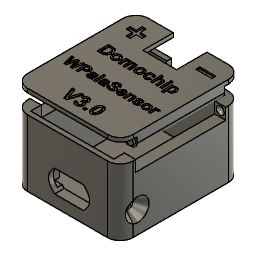
WPalaSensor v12 (Autodesk Fusion 360 design; units mm, degrees)
Autodesk Fusion 360 part; units mm, degrees
form "Form1" [no effect]
sketch "Bases" plane through (0, 0, 0) normal (0, 1, 0) x (1, 0, 0)
  line L0 (7.8348, 4.0595) -> (32.8348, 4.0595)
  line L1 (36.8348, 8.0595) -> (36.8348, 37.8595)
  line L2 (32.8348, 41.8595) -> (7.8348, 41.8595)
  line L3 (3.8348, 37.8595) -> (3.8348, 8.0595)
  arc A0 (7.8348, 41.8595) -> (3.8348, 37.8595) centre (7.8348, 37.8595) ccw
  arc A1 (36.8348, 37.8595) -> (32.8348, 41.8595) centre (32.8348, 37.8595) ccw
  arc A2 (32.8348, 4.0595) -> (36.8348, 8.0595) centre (32.8348, 8.0595) ccw
  arc A3 (3.8348, 8.0595) -> (7.8348, 4.0595) centre (7.8348, 8.0595) ccw
  arc A4 (3.8348, 8.0595) -> (7.8348, 4.0595) centre (7.8348, 8.0595) ccw
  arc A5 (32.8348, 4.0595) -> (36.8348, 8.0595) centre (32.8348, 8.0595) ccw
  line L4 (3.8348, 37.8595) -> (3.8348, 8.0595)
  line L5 (36.8348, 8.0595) -> (36.8348, 37.8595)
  line L6 (7.8348, 4.0595) -> (32.8348, 4.0595)
  arc A6 (7.8348, 41.8595) -> (3.8348, 37.8595) centre (7.8348, 37.8595) ccw
  line L7 (32.8348, 41.8595) -> (7.8348, 41.8595)
  arc A7 (36.8348, 37.8595) -> (32.8348, 41.8595) centre (32.8348, 37.8595) ccw
  line L8 (-37.5541, 37.8017) -> (-37.5541, 8.0017)
  arc A8 (-8.5541, 4.0017) -> (-4.5541, 8.0017) centre (-8.5541, 8.0017) ccw
  line L9 (-33.5541, 4.0017) -> (-8.5541, 4.0017)
  line L10 (-8.5541, 41.8017) -> (-33.5541, 41.8017)
  arc A9 (-33.5541, 41.8017) -> (-37.5541, 37.8017) centre (-33.5541, 37.8017) ccw
  arc A10 (-4.5541, 37.8017) -> (-8.5541, 41.8017) centre (-8.5541, 37.8017) ccw
  arc A11 (-37.5541, 8.0017) -> (-33.5541, 4.0017) centre (-33.5541, 8.0017) ccw
  line L11 (-4.5541, 8.0017) -> (-4.5541, 37.8017)
  line L12 (-37.5541, 36.6017) -> (-34.0541, 36.6017)
  line L13 (-34.0541, 36.6017) -> (-34.0541, 9.2017)
  line L14 (-34.0541, 9.2017) -> (-37.5541, 9.2017)
  line L15 (-37.5541, 9.2017) -> (-37.5541, 36.6017)
  line L16 (-4.5541, 36.6017) -> (-8.0541, 36.6017)
  line L17 (-8.0541, 36.6017) -> (-8.0541, 9.2017)
  line L18 (-8.0541, 9.2017) -> (-4.5541, 9.2017)
  line L19 (-4.5541, 9.2017) -> (-4.5541, 36.6017)
  dimension "d14" = 4
  dimension "d15" = 4
  dimension "d16" = 37.8
  dimension "d18" = 33
  dimension "d31" = 4
  dimension "d32" = 4
  dimension "d33" = 37.8
  dimension "d34" = 33
  dimension "d35" = 4
  dimension "d36" = 4
  dimension "d37" = 37.8
  dimension "d38" = 33
  dimension "d45" = 27.4
  dimension "d46" = 3.5
  dimension "d47" = 3.5
  constraint horizontal L0
  constraint vertical L1
  constraint horizontal L2
  constraint vertical L3
  constraint tangent L2 A0
  constraint tangent L3 A0
  constraint tangent L1 A1
  constraint tangent L2 A1
  constraint tangent L0 A2
  constraint tangent L1 A2
  constraint equal A1 A2
  constraint tangent L0 A3
  constraint tangent L3 A3
  constraint equal A1 A3
  constraint horizontal L6
  constraint vertical L5
  constraint horizontal L7
  constraint vertical L4
  constraint tangent A6 L7
  constraint tangent L4 A6
  constraint tangent L5 A7
  constraint tangent L7 A7
  constraint tangent A5 L6
  constraint tangent A5 L5
  constraint equal A5 A7
  constraint tangent A4 L6
  constraint tangent A4 L4
  constraint equal A4 A7
  constraint horizontal L9
  constraint vertical L11
  constraint horizontal L10
  constraint vertical L8
  constraint tangent L10 A9
  constraint tangent L8 A9
  constraint tangent A10 L11
  constraint tangent L10 A10
  constraint tangent A8 L9
  constraint tangent A8 L11
  constraint equal A8 A10
  constraint tangent L9 A11
  constraint tangent L8 A11
  constraint equal A10 A11
  constraint horizontal L12
  constraint vertical L13
  constraint horizontal L14
  constraint vertical L15
  constraint coincident L8 L12.start
  constraint midpoint L8 L15
  constraint horizontal L16
  constraint vertical L17
  constraint horizontal L18
  constraint vertical L19
  constraint collinear L12 L16
  constraint collinear L14 L18
  constraint collinear L11 L19
  measures "d14" radius of A0
  measures "d15" radius of A1
  measures "d16" distance of L0 L2
  measures "d18" distance of L1 L3
  measures "d31" radius of A6
  measures "d32" radius of A7
  measures "d33" distance of L6 L7
  measures "d34" distance of L4 L5
  measures "d35" radius of A9
  measures "d36" radius of A10
  measures "d37" distance of L9 L10
  measures "d38" distance of L8 L11
  measures "d45" distance of L12.end L13.end
  measures "d46" distance of L12.start L12.end
  measures "d47" distance of L16.start L16.end
extrude "Extrude1" add sketch "Bases" along normal blind 20.75 contours L0 L1 L2 L3 A0 A1 A2 A3 A4 A5 L4 L5 L6 A6 L7 A7 makes body 1
sketch "TopBox" plane through (0, 20.75, 0) normal (0, 1, 0) x (-1, 0, 0)
  arc A0 (-3.8348, -8.0595) -> (-7.8348, -4.0595) centre (-7.8348, -8.0595) ccw
  line L0 (-7.8348, -4.0595) -> (-32.8348, -4.0595)
  arc A1 (-32.8348, -4.0595) -> (-36.8348, -8.0595) centre (-32.8348, -8.0595) ccw
  line L1 (-36.8348, -8.0595) -> (-36.8348, -37.8595)
  arc A2 (-36.8348, -37.8595) -> (-32.8348, -41.8595) centre (-32.8348, -37.8595) ccw
  line L2 (-32.8348, -41.8595) -> (-7.8348, -41.8595)
  arc A3 (-7.8348, -41.8595) -> (-3.8348, -37.8595) centre (-7.8348, -37.8595) ccw
  line L3 (-3.8348, -37.8595) -> (-3.8348, -8.0595)
  line L4 (-7.3348, -5.5595) -> (-33.3348, -5.5595)
  line L5 (-33.3348, -5.5595) -> (-33.3348, -40.3595)
  line L6 (-33.3348, -40.3595) -> (-7.3348, -40.3595)
  line L7 (-7.3348, -40.3595) -> (-7.3348, -5.5595)
  line L8 (-3.8348, -37.0595) -> (-7.3348, -37.0595)
  line L9 (-7.3348, -37.0595) -> (-7.3348, -8.8595)
  line L10 (-7.3348, -8.8595) -> (-3.8348, -8.8595)
  line L11 (-3.8348, -8.8595) -> (-3.8348, -37.0595)
  line L12 (-33.3348, -37.0595) -> (-36.8348, -37.0595)
  line L13 (-36.8348, -37.0595) -> (-36.8348, -8.8595)
  line L14 (-36.8348, -8.8595) -> (-33.3348, -8.8595)
  line L15 (-33.3348, -8.8595) -> (-33.3348, -37.0595)
  dimension "d22" = 34.8
  dimension "d23" = 26
  dimension "d24" = 1.5
  dimension "d25" = 3.5
  dimension "d28" = 28.2
  constraint horizontal L4
  constraint vertical L5
  constraint horizontal L6
  constraint vertical L7
  constraint horizontal L8
  constraint vertical L9
  constraint horizontal L10
  constraint vertical L11
  constraint coincident L7 L9.end
  constraint coincident L3 L8.start
  constraint midpoint L3 L11
  constraint horizontal L12
  constraint vertical L13
  constraint horizontal L14
  constraint vertical L15
  constraint coincident L1 L13.end
  constraint coincident L5 L12.start
  constraint midpoint L1 L13
  constraint collinear L8 L12
  measures "d22" distance of L4.start L6.end
  measures "d23" distance of L4.start L4.end
  measures "d24" distance of L0 L4
  measures "d25" distance of L3 L7
  measures "d28" distance of L8.start L10.end
extrude "Extrude2" cut sketch "TopBox" against normal blind 19.5 contours L4 L5 L6 L7 L9 L15 bodies 1
extrude "Extrude3" cut sketch "TopBox" against normal blind 3.5 contours L3 L7 L8 L9 L10 L11 | L1 L5 L12 L13 L14 L15 bodies 1
extrude "Extrude4" add sketch "Bases" along normal blind 1.25 separate body contours L8 A8 L9 L10 A9 A10 A11 L11 L12 L13 L14 L16 L17 L18 | L8 L12 L13 L14 L15 | L11 L16 L17 L18 L19 makes body 2
extrude "Extrude5" add sketch "Bases" along normal blind 4.75 contours L8 L12 L13 L14 L15 | L11 L16 L17 L18 L19 bodies 2
fillet "Fillet1" radius 1.75 1 edges at (-4.5541, 4.75, -22.9017) on bodies 2
fillet "Fillet1" radius 1.75 1 edges at (-37.5541, 4.75, -22.9017) on bodies 2
sphere "SpherePrimitive10" cut diameter 2.5 placed x (1, 0, 0) y (0, 1, 0) z (0, 0, 1) at (35.0848, 19, -37.0595) bodies 1
pattern_linear "R-Pattern1" count 2 spacing 28.2 along (0, 0, 1) count 2 spacing 29.5 along (-1, 0, 0) of "SpherePrimitive10"
sphere "SpherePrimitive9" add diameter 2.5 placed x (-1, 0, 0) y (0, 1, 0) z (0, 0, -1) at (-6.3041, 3, -36.6017) bodies 2
pattern_linear "R-Pattern2" count 2 spacing 27.4 along (0, 0, 1) count 2 spacing 29.5 along (-1, 0, 0) of "SpherePrimitive9"
sketch "CutSpheres" plane through (0, 1.25, 0) normal (0, 1, 0) x (-1, 0, 0)
  line L0 (8.0541, -36.6017) -> (4.5541, -36.6017)
  line L1 (4.5541, -36.6017) -> (4.5541, -37.8017)
  arc A0 (4.5541, -37.8017) -> (8.5541, -41.8017) centre (8.5541, -37.8017) ccw
  line L2 (8.5541, -41.8017) -> (33.5541, -41.8017)
  arc A1 (33.5541, -41.8017) -> (37.5541, -37.8017) centre (33.5541, -37.8017) ccw
  line L3 (37.5541, -37.8017) -> (37.5541, -36.6017)
  line L4 (37.5541, -36.6017) -> (34.0541, -36.6017)
  line L5 (34.0541, -36.6017) -> (34.0541, -9.2017)
  line L6 (34.0541, -9.2017) -> (37.5541, -9.2017)
  line L7 (37.5541, -9.2017) -> (37.5541, -8.0017)
  arc A2 (37.5541, -8.0017) -> (33.5541, -4.0017) centre (33.5541, -8.0017) ccw
  line L8 (33.5541, -4.0017) -> (8.5541, -4.0017)
  arc A3 (8.5541, -4.0017) -> (4.5541, -8.0017) centre (8.5541, -8.0017) ccw
  line L9 (4.5541, -8.0017) -> (4.5541, -9.2017)
  line L10 (4.5541, -9.2017) -> (8.0541, -9.2017)
  line L11 (8.0541, -9.2017) -> (8.0541, -36.6017)
  line L12 (7.5541, -37.8517) -> (5.0541, -37.8517)
  line L13 (5.0541, -37.8517) -> (5.0541, -37.1517)
  line L14 (5.0541, -37.1517) -> (7.5541, -37.1517)
  line L15 (7.5541, -37.1517) -> (7.5541, -37.8517)
  line L16 (4.5541, -8.0017) -> (4.5541, -37.8017)
  line L17 (4.5541, -36.6017) -> (8.0541, -36.6017)
  line L18 (7.5541, -8.6517) -> (5.0541, -8.6517)
  line L19 (5.0541, -8.6517) -> (5.0541, -7.9517)
  line L20 (5.0541, -7.9517) -> (7.5541, -7.9517)
  line L21 (7.5541, -7.9517) -> (7.5541, -8.6517)
  line L22 (37.0541, -8.6517) -> (34.5541, -8.6517)
  line L23 (34.5541, -8.6517) -> (34.5541, -7.9517)
  line L24 (34.5541, -7.9517) -> (37.0541, -7.9517)
  line L25 (37.0541, -7.9517) -> (37.0541, -8.6517)
  line L26 (37.0541, -37.8517) -> (34.5541, -37.8517)
  line L27 (34.5541, -37.8517) -> (34.5541, -37.1517)
  line L28 (34.5541, -37.1517) -> (37.0541, -37.1517)
  line L29 (37.0541, -37.1517) -> (37.0541, -37.8517)
  line L30 (8.0541, -9.2017) -> (4.5541, -9.2017)
  line L31 (34.0541, -9.2017) -> (37.5541, -9.2017)
  line L32 (37.5541, -36.6017) -> (34.0541, -36.6017)
  line L33 (37.5541, -37.8017) -> (37.5541, -8.0017)
  dimension "d71" = 0.5
  dimension "d72" = 2.5
  dimension "d73" = 0.55
  dimension "d74" = 0.7
  dimension "d77" = 0.55
  dimension "d78" = 0.55
  dimension "d79" = 0.55
  dimension "d80" = 0.7
  dimension "d81" = 0.7
  dimension "d82" = 0.7
  dimension "d83" = 0.5
  dimension "d84" = 0.5
  dimension "d85" = 0.5
  dimension "d86" = 2.5
  dimension "d87" = 2.5
  dimension "d88" = 2.5
  constraint horizontal L12
  constraint vertical L13
  constraint horizontal L14
  constraint vertical L15
  constraint horizontal L18
  constraint vertical L19
  constraint horizontal L20
  constraint vertical L21
  constraint horizontal L22
  constraint vertical L23
  constraint horizontal L24
  constraint vertical L25
  constraint horizontal L26
  constraint vertical L27
  constraint horizontal L28
  constraint vertical L29
  measures "d71" distance of L13 L16
  measures "d72" distance of L12.start L12.end
  measures "d73" distance of L14 L17
  measures "d74" distance of L12.end L13.end
  measures "d77" distance of L18 L30
  measures "d78" distance of L22 L31
  measures "d79" distance of L28 L32
  measures "d80" distance of L18.end L19.end
  measures "d81" distance of L22.start L24.end
  measures "d82" distance of L26.start L28.end
  measures "d83" distance of L16 L19
  measures "d84" distance of L25 L33
  measures "d85" distance of L29 L33
  measures "d86" distance of L26.start L26.end
  measures "d87" distance of L23.end L24.end
  measures "d88" distance of L19.end L20.end
extrude "Extrude6" cut sketch "CutSpheres" along normal blind 3 contours L12 L13 L14 L15 | L18 L19 L20 L21 | L22 L23 L24 L25 | L26 L27 L28 L29 bodies 2
sketch "Supports" plane through (0, 1.25, 0) normal (0, 1, 0) x (-1, 0, 0)
  line L0 (-7.3348, -40.3595) -> (-7.3348, -5.5595)
  line L1 (-7.3348, -5.5595) -> (-33.3348, -5.5595)
  line L2 (-33.3348, -5.5595) -> (-33.3348, -40.3595)
  line L3 (-33.3348, -40.3595) -> (-7.3348, -40.3595)
  line L4 (-7.3348, -5.5595) -> (-10.3348, -5.5595)
  line L5 (-10.3348, -5.5595) -> (-10.3348, -11.5595)
  line L6 (-10.3348, -11.5595) -> (-7.3348, -11.5595)
  line L7 (-7.3348, -11.5595) -> (-7.3348, -5.5595)
  line L8 (-7.3348, -40.3595) -> (-10.3348, -40.3595)
  line L9 (-10.3348, -40.3595) -> (-10.3348, -34.3595)
  line L10 (-10.3348, -34.3595) -> (-7.3348, -34.3595)
  line L11 (-7.3348, -34.3595) -> (-7.3348, -40.3595)
  line L12 (-33.3348, -40.3595) -> (-30.3348, -40.3595)
  line L13 (-30.3348, -40.3595) -> (-30.3348, -34.3595)
  line L14 (-30.3348, -34.3595) -> (-33.3348, -34.3595)
  line L15 (-33.3348, -34.3595) -> (-33.3348, -40.3595)
  line L16 (-33.3348, -5.5595) -> (-28.3348, -5.5595)
  line L17 (-28.3348, -5.5595) -> (-28.3348, -11.5595)
  line L18 (-28.3348, -11.5595) -> (-33.3348, -11.5595)
  line L19 (-33.3348, -11.5595) -> (-33.3348, -5.5595)
  line L20 (-28.3348, -5.5595) -> (-10.3348, -5.5595)
  line L21 (-10.3348, -5.5595) -> (-10.3348, -7.0595)
  line L22 (-10.3348, -7.0595) -> (-28.3348, -7.0595)
  line L23 (-28.3348, -7.0595) -> (-28.3348, -5.5595)
  dimension "d93" = 6
  dimension "d94" = 3
  dimension "d95" = 6
  dimension "d96" = 6
  dimension "d97" = 3
  dimension "d98" = 3
  dimension "d143" = 6
  dimension "d144" = 5
  dimension "d145" = 1.5
  constraint horizontal L4
  constraint vertical L5
  constraint horizontal L6
  constraint vertical L7
  constraint coincident L0.end L1.start
  constraint horizontal L8
  constraint vertical L9
  constraint horizontal L10
  constraint vertical L11
  constraint coincident L0.start L3.end
  constraint horizontal L12
  constraint vertical L13
  constraint horizontal L14
  constraint vertical L15
  constraint coincident L2.end L3.start
  constraint horizontal L16
  constraint vertical L17
  constraint horizontal L18
  constraint vertical L19
  constraint coincident L1.end L2.start
  constraint horizontal L20
  constraint vertical L21
  constraint horizontal L22
  constraint vertical L23
  constraint coincident L5 L21.end
  measures "d93" distance of L4.end L5.end
  measures "d94" distance of L5.end L6.end
  measures "d95" distance of L8.end L9.end
  measures "d96" distance of L12.end L13.end
  measures "d97" distance of L0.start L8.end
  measures "d98" distance of L2.end L12.end
  measures "d143" distance of L16.end L17.end
  measures "d144" distance of L17.end L18.end
  measures "d145" distance of L20 L22
extrude "Extrude7" add sketch "Supports" along normal blind 3 contours L0 L3 L8 L9 L10 L11 | L0 L1 L4 L5 L6 L7 L21 | L2 L3 L12 L13 L14 L15 | L1 L5 L17 L20 L21 L22 L23 | L1 L2 L16 L17 L18 L19 L23 bodies 1
sketch "ResetHole" plane through (36.8348, 0, 0) normal (1, 0, 0) x (0, 0, -1)
  line L0 (8.8595, 17.25) -> (8.8595, 20.75)
  line L1 (8.0595, 20.75) -> (8.0595, 0)
  line L2 (8.0595, 0) -> (37.8595, 0)
  line L3 (37.8595, 0) -> (37.8595, 20.75)
  line L4 (37.0595, 20.75) -> (37.0595, 17.25)
  line L5 (37.0595, 17.25) -> (8.8595, 17.25)
  circle A0 centre (9.5595, 6.85) radius 1.5
  line L6 (8.0595, 0) -> (37.8595, 0)
  line L7 (8.8595, 20.75) -> (8.0595, 20.75)
  line L8 (37.8595, 20.75) -> (37.0595, 20.75)
  dimension "d101" = 1.5
  dimension "d102" = 3
  dimension "d103" = 6.85
  measures "d101" distance of L1 A0.centre
  measures "d102" diameter of A0
  measures "d103" distance of A0.centre L6
extrude "Extrude8" cut sketch "ResetHole" against normal blind 3.5 contours A0 bodies 1
chamfer "Chamfer3" distance 2 distance2 3 1 edges at (36.8348, 7.3924, -8.161) measured on face at (36.8348, 8.1079, -28.6539) on bodies 1
sketch "USBHole" plane through (0, 0, -4.0595) normal (0, 0, 1) x (1, 0, 0)
  line L0 (7.8348, 0) -> (32.8348, 0)
  line L1 (32.8348, 0) -> (32.8348, 20.75)
  line L2 (32.8348, 20.75) -> (7.8348, 20.75)
  line L3 (7.8348, 20.75) -> (7.8348, 0)
  line L4 (16.3348, 10.55) -> (25.3348, 10.55)
  line L5 (25.3348, 3.55) -> (16.3348, 3.55)
  spline S0 degree 5 poles (16.3348, 10.55) (16.188, 10.41) (15.907, 10.13) (15.5241, 9.71) (15.0918, 9.15) (14.6906, 8.45) (14.4412, 7.75) (14.3558, 7.05) (14.4412, 6.35) (14.6906, 5.65) (15.0918, 4.95) (15.5241, 4.39) (15.907, 3.97) (16.188, 3.69) (16.3348, 3.55) knots 0 0 0 0 0 0 0.1 0.2 0.3 0.4 0.5 0.6 0.7 0.8 0.9 1 1 1 1 1 1
  spline S1 degree 5 poles (25.3348, 3.55) (25.4817, 3.69) (25.7626, 3.97) (26.1456, 4.39) (26.5779, 4.95) (26.979, 5.65) (27.2285, 6.35) (27.3139, 7.05) (27.2285, 7.75) (26.979, 8.45) (26.5779, 9.15) (26.1456, 9.71) (25.7626, 10.13) (25.4817, 10.41) (25.3348, 10.55) knots 0 0 0 0 0 0 0.1 0.2 0.3 0.4 0.5 0.6 0.7 0.8 0.9 1 1 1 1 1 1
  line L6 (16.3348, 10.55) -> (16.3348, 3.55)
  line L7 (25.3348, 10.55) -> (25.3348, 3.55)
  line L8 (7.8348, 3.55) -> (32.8348, 3.55)
  line L9 (7.8348, 0) -> (32.8348, 0)
  point P0 (14.3983, 7.05)
  point P1 (14.3983, 7.05)
  point P2 (27.2713, 7.05)
  point P3 (27.2713, 7.05)
  point P4 (20.3348, 3.55)
  dimension "d104" = 9
  dimension "d105" = 7
  dimension "d106" = 4
  dimension "d107" = 4
  dimension "d108" = 4
  dimension "d109" = 4
  dimension "d115" = 7.05
  dimension "d138" = 4
  constraint horizontal L4
  constraint parallel L4 L5
  constraint coincident P1 P0
  constraint coincident P3 P2
  constraint perpendicular L5 L7
  constraint parallel L6 L7
  constraint coincident L3 L8.start
  constraint coincident L1 L8.end
  constraint perpendicular L1 L8
  constraint coincident L8 P4
  constraint midpoint L8 P4
  constraint coincident L5.end L8
  measures "d104" distance of L4.start L4.end
  measures "d105" distance of L4.end L5.start
  measures "d106" distance of L4.start P1
  measures "d107" distance of L5.end P1
  measures "d108" distance of L4.end P3
  measures "d109" distance of L5.start P3
  measures "d115" distance of P1 L9
  measures "d138" distance of L5.end P4
extrude "Extrude9" cut sketch "USBHole" against normal blind 3 contours L4 L5 L6 L7 L8 | S0 L6 | S1 L7 bodies 1
sketch "BornierHole" plane through (0, 0, -41.8595) normal (0, 0, -1) x (-1, 0, 0)
  line L0 (-32.8348, 0) -> (-7.8348, 0)
  line L1 (-7.8348, 0) -> (-7.8348, 20.75)
  line L2 (-7.8348, 20.75) -> (-32.8348, 20.75)
  line L3 (-32.8348, 20.75) -> (-32.8348, 0)
  line L4 (-25.5848, 20.75) -> (-15.0848, 20.75)
  line L5 (-15.0848, 20.75) -> (-15.0848, 18.25)
  line L6 (-15.0848, 18.25) -> (-25.5848, 18.25)
  line L7 (-25.5848, 18.25) -> (-25.5848, 20.75)
  dimension "d116" = 10.5
  dimension "d147" = 18.25
  constraint horizontal L4
  constraint vertical L5
  constraint horizontal L6
  constraint vertical L7
  constraint coincident L2 L4.start
  constraint midpoint L2 L4
  measures "d116" distance of L4.start L4.end
  measures "d147" distance of L0 L6
extrude "Extrude10" cut sketch "BornierHole" against normal blind 1.5 contours L2 L4 L5 L6 L7 bodies 1
sketch "BordnierHoleAndMaintainLeg" plane through (0, 1.25, 0) normal (0, 1, 0) x (-1, 0, 0)
  line L0 (8.0541, -36.6017) -> (4.5541, -36.6017)
  line L1 (4.5541, -36.6017) -> (4.5541, -37.8017)
  arc A0 (4.5541, -37.8017) -> (8.5541, -41.8017) centre (8.5541, -37.8017) ccw
  line L2 (8.5541, -41.8017) -> (33.5541, -41.8017)
  arc A1 (33.5541, -41.8017) -> (37.5541, -37.8017) centre (33.5541, -37.8017) ccw
  line L3 (37.5541, -37.8017) -> (37.5541, -36.6017)
  line L4 (37.5541, -36.6017) -> (34.0541, -36.6017)
  line L5 (34.0541, -36.6017) -> (34.0541, -9.2017)
  line L6 (34.0541, -9.2017) -> (37.5541, -9.2017)
  line L7 (37.5541, -9.2017) -> (37.5541, -8.0017)
  arc A2 (37.5541, -8.0017) -> (33.5541, -4.0017) centre (33.5541, -8.0017) ccw
  line L8 (33.5541, -4.0017) -> (8.5541, -4.0017)
  arc A3 (8.5541, -4.0017) -> (4.5541, -8.0017) centre (8.5541, -8.0017) ccw
  line L9 (4.5541, -8.0017) -> (4.5541, -9.2017)
  line L10 (4.5541, -9.2017) -> (8.0541, -9.2017)
  line L11 (8.0541, -9.2017) -> (8.0541, -36.6017)
  line L12 (26.8041, -41.8017) -> (16.3041, -41.8017)
  line L13 (16.3041, -41.8017) -> (16.3041, -32.3017)
  line L14 (16.3041, -32.3017) -> (26.8041, -32.3017)
  line L15 (26.8041, -32.3017) -> (26.8041, -41.8017)
  line L16 (29.0541, -15.3017) -> (13.0541, -15.3017)
  line L17 (13.0541, -15.3017) -> (13.0541, -13.3017)
  line L18 (13.0541, -13.3017) -> (29.0541, -13.3017)
  line L19 (29.0541, -13.3017) -> (29.0541, -15.3017)
  line L20 (37.5541, -36.6017) -> (37.5541, -9.2017)
  line L21 (4.5541, -9.2017) -> (4.5541, -36.6017)
  point P0 (21.0541, -41.8017)
  point P1 (21.5541, -41.8017)
  dimension "d120" = 10.5
  dimension "d121" = 9.5
  dimension "d149" = 0.5
  dimension "d150" = 2
  dimension "d151" = 8.5
  dimension "d152" = 8.5
  dimension "d153" = 28.5
  constraint horizontal L12
  constraint vertical L13
  constraint horizontal L14
  constraint vertical L15
  constraint coincident L2 L12.start
  constraint midpoint L2 P0
  constraint midpoint L12 P1
  constraint horizontal L16
  constraint vertical L17
  constraint horizontal L18
  constraint vertical L19
  measures "d120" distance of L12.start L12.end
  measures "d121" distance of L12.start L14.end
  measures "d149" distance of P0 P1
  measures "d150" distance of L16.end L17.end
  measures "d151" distance of L19 L20
  measures "d152" distance of L17 L21
  measures "d153" distance of L2 L18
extrude "Extrude11" cut sketch "BordnierHoleAndMaintainLeg" against normal blind 1.25 contours L2 L12 L13 L14 L15 bodies 2
extrude "Extrude14" add sketch "BordnierHoleAndMaintainLeg" along normal blind 2 contours L16 L17 L18 L19 bodies 2
chamfer "Chamfer4" distance 2 angle 45 2 edges at (-13.0541, 3.25, -14.3017) (-29.0541, 3.25, -14.3017) on bodies 2
sketch "ModuleName" plane through (0, 0, 0) normal (0, -1, 0) x (1, 0, 0)
  line L0 (-26.8041, -41.8017) -> (-26.8041, -32.3017)
  line L1 (-26.8041, -32.3017) -> (-16.3041, -32.3017)
  line L2 (-16.3041, -32.3017) -> (-16.3041, -41.8017)
  line L3 (-16.3041, -41.8017) -> (-8.5541, -41.8017)
  arc A0 (-8.5541, -41.8017) -> (-4.5541, -37.8017) centre (-8.5541, -37.8017) ccw
  line L4 (-4.5541, -37.8017) -> (-4.5541, -8.0017)
  arc A1 (-4.5541, -8.0017) -> (-8.5541, -4.0017) centre (-8.5541, -8.0017) ccw
  line L5 (-8.5541, -4.0017) -> (-33.5541, -4.0017)
  arc A2 (-33.5541, -4.0017) -> (-37.5541, -8.0017) centre (-33.5541, -8.0017) ccw
  line L6 (-37.5541, -8.0017) -> (-37.5541, -37.8017)
  arc A3 (-37.5541, -37.8017) -> (-33.5541, -41.8017) centre (-33.5541, -37.8017) ccw
  line L7 (-33.5541, -41.8017) -> (-26.8041, -41.8017)
  line L8 (-7.9291, -36.6639) -> (-12.9291, -36.6639)
  line L9 (-12.9291, -36.6639) -> (-12.9291, -35.4639)
  line L10 (-12.9291, -35.4639) -> (-7.9291, -35.4639)
  line L11 (-7.9291, -35.4639) -> (-7.9291, -36.6639)
  line L12 (-9.8291, -38.5639) -> (-11.0291, -38.5639)
  line L13 (-11.0291, -38.5639) -> (-11.0291, -33.5639)
  line L14 (-11.0291, -33.5639) -> (-9.8291, -33.5639)
  line L15 (-9.8291, -33.5639) -> (-9.8291, -38.5639)
  line L16 (-29.6791, -36.6639) -> (-34.6791, -36.6639)
  line L17 (-34.6791, -36.6639) -> (-34.6791, -35.4639)
  line L18 (-34.6791, -35.4639) -> (-29.6791, -35.4639)
  line L19 (-29.6791, -35.4639) -> (-29.6791, -36.6639)
  line L20 (-4.5541, -33.5639) -> (-16.3041, -33.5639)
  line L21 (-26.8041, -35.4639) -> (-37.5541, -35.4639)
  line L22 (-15.4308, -24.0017) -> (-26.6774, -24.0017) construction
  line L23 (-26.6774, -24.0017) -> (-26.6774, -29.4655) construction
  line L24 (-26.6774, -29.4655) -> (-15.4308, -29.4655) construction
  line L25 (-15.4308, -29.4655) -> (-15.4308, -24.0017) construction
  line L26 (-15.0541, -16.0017) -> (-27.0541, -16.0017) construction
  line L27 (-27.0541, -16.0017) -> (-27.0541, -20.0497) construction
  line L28 (-27.0541, -20.0497) -> (-15.0541, -20.0497) construction
  line L29 (-15.0541, -20.0497) -> (-15.0541, -16.0017) construction
  line L30 (-16.5541, -6.5017) -> (-25.5541, -6.5017) construction
  line L31 (-25.5541, -6.5017) -> (-25.5541, -11.5497) construction
  line L32 (-25.5541, -11.5497) -> (-16.5541, -11.5497) construction
  line L33 (-16.5541, -11.5497) -> (-16.5541, -6.5017) construction
  line L34 (-4.5541, -24.0017) -> (-37.5541, -24.0017)
  line L35 (-4.5541, -16.0017) -> (-37.5541, -16.0017)
  line L36 (-4.5541, -6.5017) -> (-37.5541, -6.5017)
  dimension "d157" = 1.2
  dimension "d158" = 5
  dimension "d159" = 1.9
  dimension "d160" = 1.9
  dimension "d161" = 5
  dimension "d162" = 1.2
  dimension "d164" = 3.5
  dimension "d165" = 3.2
  dimension "d166" = 4
  dimension "d167" = 2.5
  dimension "d168" = 12
  dimension "d169" = 20
  text T0 "Domochip" font "Arial" height 3.5 bold align centre middle in box 11.2466 x 5.4639 at (-15.4308, -24.0017) x (-1, 0) y (0, -1) spacing 1 kerned
  text T1 "WPalaSensor" font "Arial" height 3.2 bold align centre middle in box 12 x 4.048 at (-15.0541, -16.0017) x (-1, 0) y (0, -1) spacing 1 kerned
  text T2 "V3.0" font "Arial" height 4 bold align centre middle in box 9 x 5.048 at (-16.5541, -6.5017) x (-1, 0) y (0, -1) spacing 1 kerned
  constraint horizontal L8
  constraint vertical L9
  constraint horizontal L10
  constraint vertical L11
  constraint horizontal L12
  constraint vertical L13
  constraint horizontal L14
  constraint vertical L15
  constraint equal L8 L15
  constraint equal L11 L12
  constraint horizontal L16
  constraint vertical L17
  constraint horizontal L18
  constraint vertical L19
  constraint collinear L10 L18
  constraint coincident L4 L20.start
  constraint coincident L2 L20.end
  constraint perpendicular L2 L20
  constraint midpoint L14 L20
  constraint coincident L0 L21.start
  constraint coincident L6 L21.end
  constraint perpendicular L6 L21
  constraint midpoint L18 L21
  constraint coincident L4 L34.start
  constraint coincident L6 L34.end
  constraint perpendicular L6 L34
  constraint coincident L4 L35.start
  constraint coincident L6 L35.end
  constraint perpendicular L6 L35
  constraint coincident L4 L36.start
  constraint coincident L6 L36.end
  constraint perpendicular L6 L36
  constraint collinear L30 L36
  constraint collinear L26 L35
  constraint collinear L22 L34
  constraint midpoint L22 L34
  constraint midpoint L26 L35
  constraint midpoint L30 L36
  measures "d157" distance of L8.start L10.end
  measures "d158" distance of L8.start L8.end
  measures "d159" distance of L11 L15
  measures "d160" distance of L8 L12
  measures "d161" distance of L16.start L16.end
  measures "d162" distance of L16.start L18.end
  measures "d167" distance of L5 L36
  measures "d168" distance of L5 L35
  measures "d169" distance of L5 L34
extrude "Extrude13" cut sketch "ModuleName" sketch "ModuleName" against normal blind 0.5 contours L16 L17 L18 L19 L21 | L10 L13 L14 L15 L20 | L8 L9 L10 L13 | L8 L10 L13 L15 | L8 L10 L11 L15 | L8 L12 L13 L15 of sketch 2 text T0 T1 T2 bodies 2
move_body "Move1" bodies 2 to x (-1, 0, 0) y (0, -1, 0) z (0, 0, 1) at (-0.6081, 28, 0)
equation "_width = 34.8 mm" comment "width of the box (affects the length of the hinges)"
equation "_length = 26 mm" comment "length of the box"
equation "_height = 19.5 mm" comment "height of the box"
equation "_rounding = 4 mm" comment "rounding radius of the corners of the box"
equation "_minimumWallThickness = 0.5 mm" comment "thickness of the walls around the magnets"
equation "_sidewallThickness = 1.5 mm" comment "thickness of the side walls without the hinge"
equation "_horizontalThickness = 1.25 mm" comment "thickness of the bottom of the box or the top of the lid"
equation "_magnetDiameter = 2.5 mm" comment "diameter of magnets in the hinge"
equation "_magnetHeight = 1 mm" comment "height magnets in the hinge"
equation "_hingeGap = 0.4 mm" comment "gap bewteen the lid and box parts"
equation "_hingeOverlap = 0.15 mm" comment "Size of lid's spheres that go into box holes"
equation "d14 = _rounding"
equation "d15 = _rounding"
equation "d16 = _width + 2 * _sidewallThickness"
equation "d18 = _length + 4 * _minimumWallThickness + 2 * _magnetDiameter"
equation "d20 = _height + _horizontalThickness"
equation "d22 = _width"
equation "d23 = _length"
equation "d24 = _sidewallThickness"
equation "d25 = 2 * _minimumWallThickness + _magnetDiameter"
equation "d26 = -_height"
equation "d28 = _width + 2 * _sidewallThickness - 2 * _rounding - 2 * _magnetHeight + _hingeGap"
equation "d29 = -_magnetDiameter - 2 * _minimumWallThickness"
equation "d31 = _rounding"
equation "d32 = _rounding"
equation "d33 = _width + 2 * _sidewallThickness"
equation "d34 = _length + 4 * _minimumWallThickness + 2 * _magnetDiameter"
equation "d35 = _rounding"
equation "d36 = _rounding"
equation "d37 = _width + 2 * _sidewallThickness"
equation "d38 = _length + 4 * _minimumWallThickness + 2 * _magnetDiameter"
equation "d43 = _horizontalThickness"
equation "d45 = _width + 2 * _sidewallThickness - 2 * _rounding - 2 * _magnetHeight - _hingeGap"
equation "d46 = _magnetDiameter + 2 * _minimumWallThickness"
equation "d47 = _magnetDiameter + 2 * _minimumWallThickness"
equation "d48 = _horizontalThickness + _magnetDiameter + 2 * _minimumWallThickness"
equation "d50 = ( _magnetDiameter + 2 * _minimumWallThickness ) / 2"
equation "d51 = ( _magnetDiameter + 2 * _minimumWallThickness ) / 2"
equation "d59 = _width + 2 * _sidewallThickness - 2 * _rounding - 2 * _magnetHeight + _hingeGap"
equation "d60 = -_length - _magnetDiameter - 2 * _minimumWallThickness"
equation "d64 = _width + 2 * _sidewallThickness - 2 * _rounding - 2 * _magnetHeight - _hingeGap"
equation "d65 = -_length - _magnetDiameter - 2 * _minimumWallThickness"
equation "d71 = _minimumWallThickness"
equation "d72 = _magnetDiameter"
equation "d73 = _hingeGap + _hingeOverlap"
equation "d74 = _magnetDiameter / 2 - _hingeGap - _hingeOverlap"
equation "d75 = _minimumWallThickness + _magnetDiameter"
equation "d77 = _hingeGap + _hingeOverlap"
equation "d78 = _hingeGap + _hingeOverlap"
equation "d79 = _hingeGap + _hingeOverlap"
equation "d80 = _magnetDiameter / 2 - _hingeGap - _hingeOverlap"
equation "d81 = _magnetDiameter / 2 - _hingeGap - _hingeOverlap"
equation "d82 = _magnetDiameter / 2 - _hingeGap - _hingeOverlap"
equation "d83 = _minimumWallThickness"
equation "d84 = _minimumWallThickness"
equation "d85 = _minimumWallThickness"
equation "d86 = _magnetDiameter"
equation "d87 = _magnetDiameter"
equation "d88 = _magnetDiameter"
equation "d101 = 4 mm - _rounding + _sidewallThickness"
equation "d103 = _horizontalThickness + 3 mm + 1.6 mm + 1 mm"
equation "d111 = -_magnetDiameter - 2 * _minimumWallThickness"
equation "d115 = 3 mm + 2.8 mm + _horizontalThickness"
equation "d118 = -_sidewallThickness"
equation "d121 = 8 mm + _sidewallThickness"
equation "d127 = -_horizontalThickness"
equation "d137 = _magnetDiameter"
equation "d146 = _magnetDiameter"
equation "d147 = 17 mm + _horizontalThickness"
equation "d151 = 5 mm + 2 * _minimumWallThickness + _magnetDiameter"
equation "d152 = 5 mm + 2 * _minimumWallThickness + _magnetDiameter"
equation "d153 = 27 mm + _sidewallThickness"
named bodies: "WPalaSensor Box", "WPalaSensor Lid"
